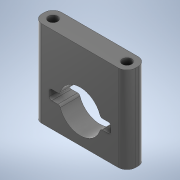
# Autodesk Inventor part: inner_mount
Saved by Autodesk Inventor 2020 (Build 240168000, 168)
## iProperties
Created: 2024-02-03
Part Number: inner_mount
Material: Пластик АБС
Document SubType Name: Modeling
Designer: 4s
Density: 1.06 g/cm^3
Appearance: Гладкая — черная
Author: 4s
Autodesk Inventor part; units mm, degrees
ref_plane "YZ Plane" through (0, 0, 0) normal (1, 0, 0) x (0, 1, 0)
ref_plane "XZ Plane" through (0, 0, 0) normal (0, 1, 0) x (-1, 0, 0)
ref_plane "XY Plane" through (0, 0, 0) normal (0, 0, 1) x (1, 0, 0)
sketch "Эскиз1" plane through (0, 0, 0) normal (1, 0, 0) x (0, 1, 0)
  point P0 (0, 0)
sketch "Эскиз2" plane through (0, 0, 0) normal (0, 1, 0) x (-1, 0, 0)
  line L0 (19, -4) -> (-19, -4)
  line L1 (-19, -4) -> (-19, 4)
  line L2 (-19, 4) -> (19, 4)
  line L3 (19, 4) -> (19, -4)
  line L4 (19, -4) -> (-19, 4) construction
  line L5 (-19, -4) -> (19, 4) construction
  line L6 (19, 0) -> (-19, 0) construction
  circle A0 centre (-15, 0) radius 1.9
  line L7 (0, -4) -> (0, 4) construction
  circle A1 centre (15, 0) radius 1.9
  point P0 (0, 0)
  dimension "d1" = 30
  dimension "d2" = 3.8
  dimension "d3" = 38
  dimension "d4" = 8
  constraints: 16 end point, 6 midpoint, 2 centre point, 2 parallel, 1 horizontal, 1 perpendicular, 1 point on line, 1 symmetric about line, 1 other
  measures "d1" distance of A0.centre A1.centre
  measures "d2" diameter of A0
  measures "d3" distance of L1.end L2.end
  measures "d4" distance between parallel lines of L2 L0
extrude "Выдавливание1" add sketch "Эскиз2" along normal blind 35
fillet "Сопряжение1" radius 3.5 4 edges at (19, 17.5, 4) (19, 17.5, -4) (-19, 17.5, 4) (-19, 17.5, -4)
sketch "Эскиз3" plane through (-15.5, 0, 4) normal (0, 0, 1) x (1, 0, 0)
  line L0 (28.6, 35) -> (28.6, 0) construction
  line L1 (0, 0) -> (0, 35) construction
  line L2 (0, 0) -> (31, 0) construction
  line L3 (31, 35) -> (31, 0) construction
  line L4 (0, 35) -> (31, 35) construction
  line L5 (32.4, 35) -> (32.4, 0) construction
  line L6 (34.5, 35) -> (31, 35) construction
  line L7 (31, 35) -> (31, 0) construction
  line L8 (31, 0) -> (34.5, 0) construction
  line L9 (34.5, 0) -> (34.5, 35) construction
  line L10 (-1.4, 35) -> (-1.4, 0) construction
  line L11 (0, 35) -> (-3.5, 35) construction
  line L12 (-3.5, 35) -> (-3.5, 0) construction
  line L13 (-3.5, 0) -> (0, 0) construction
  line L14 (0, 0) -> (0, 35) construction
  line L15 (0, 0) -> (0, 35) construction
  line L16 (-1.4, 35) -> (2.4, 35) construction
  line L17 (28.6, 35) -> (32.4, 35) construction
  line L18 (28.6, 0) -> (32.4, 0) construction
  line L19 (-1.4, 35) -> (2.4, 35) construction
  line L20 (-1.4, 0) -> (2.4, 0) construction
  line L21 (-1.4, 35) -> (2.4, 35) construction
  line L22 (-1.4, 0) -> (2.4, 0) construction
  line L23 (2.4, 35) -> (2.4, 0) construction
  line L24 (28.6, 35) -> (2.4, 0) construction
  line L25 (2.4, 35) -> (28.6, 0) construction
  line L26 (15.5, 17.5) -> (15.5, 35) construction
  line L27 (0, 35) -> (31, 35) construction
  circle A0 centre (15.5, 12) radius 8.5
  point P0 (15.5, 0)
  dimension "d8" = 17
  dimension "d9" = 12
  constraints: 6 end point, 1 centre point, 1 midpoint, 1 point on line, 2 other
  measures "d8" diameter of A0
  measures "d9" distance of point (15.5, 0) A0.centre
extrude "Выдавливание2" cut sketch "Эскиз3" against normal blind 35
sketch "Эскиз4" plane through (-15.5, 0, 4) normal (0, 0, 1) x (1, 0, 0)
  circle A0 centre (15.5, 12) radius 8.5 projected
  line L0 (0, 0) -> (0, 35) construction
  line L1 (0, 0) -> (31, 0) construction
  line L2 (31, 35) -> (31, 0) construction
  line L3 (0, 35) -> (31, 35) construction
  line L4 (23.7614, 14) -> (28, 14)
  line L5 (28, 14) -> (28, 10)
  line L6 (28, 10) -> (23.7614, 10)
  line L7 (24, 10) -> (24, 14) construction
  circle A1 centre (15.5, 12) radius 8.5 construction
  line L8 (7, 12) -> (24, 12) construction
  line L9 (15.5, 12) -> (15.5, 20.5) construction
  line L10 (7.2386, 14) -> (3, 14)
  line L11 (3, 14) -> (3, 10)
  line L12 (3, 10) -> (7.2386, 10)
  point P0 (15.5, 0)
  dimension "d13" = 4
  dimension "d14" = 4
  constraints: 18 end point, 5 point on circle, 4 symmetric about line, 2 horizontal, 2 midpoint, 2 parallel, 2 point on line, 1 coincident, 1 perpendicular, 1 vertical, 1 other
  measures "d13" distance of L4.end L5.end
  measures "d14" distance from line of point (24, 12) L5
extrude "Выдавливание3" cut sketch "Эскиз4" against normal blind 10 contours A0 L4 L5 L6 | A0 L12 L11 L10
fillet "Сопряжение2" radius 1 8 edges at (-12.5, 14, 0) (-12.5, 10, 0) (-8.2614, 14, 0) (-8.2614, 10, 0) (8.2614, 14, 0) (8.2614, 10, 0) (12.5, 10, 0) (12.5, 14, 0)
